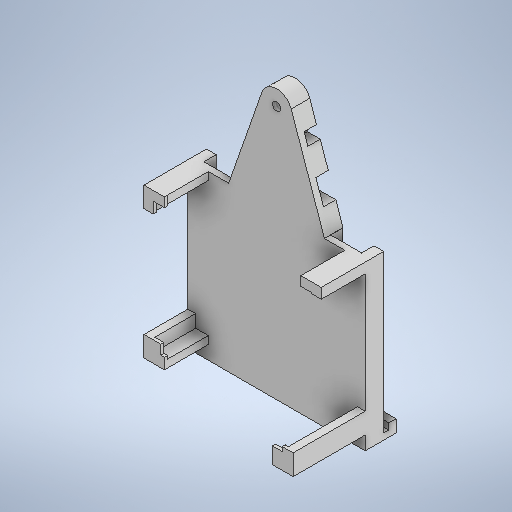
# Autodesk Inventor part: SEN5X_Mount
Saved by Autodesk Inventor 2025 (Build 290162010, 162A)
## iProperties
Created: 2024-07-08
Part Number: SEN5X_Mount
Material: Generic
Document SubType Name: Modeling
Designer: vncnt
Density: 1 g/cm^3
Appearance: Default
Author: vncnt
## iProperties of the stored document SEN5X_Mount_3DPrint.ipt
Created: 2024-07-08
Part Number: SEN5X_Mount_3DPrint
Material: Generic
Document SubType Name: Modeling
Designer: vncnt
Density: 1 g/cm^3
Appearance: Default
Author: vncnt
Autodesk Inventor part; units mm, degrees
ref_plane "YZ Plane" through (0, 0, 0) normal (1, 0, 0) x (0, 1, 0)
ref_plane "XZ Plane" through (0, 0, 0) normal (0, 1, 0) x (-1, 0, 0)
ref_plane "XY Plane" through (0, 0, 0) normal (0, 0, 1) x (1, 0, 0)
sketch "Sketch1" plane through (0, 0, 0) normal (0, 0, 1) x (1, 0, 0)
  line L0 (-28.65, -41.095) -> (28.65, -41.095)
  line L1 (28.65, -41.095) -> (28.65, 11.845)
  line L2 (-28.65, 11.755) -> (-28.65, -41.095)
  line L3 (-28.65, -41.095) -> (28.65, 41.095) construction
  line L4 (28.65, -41.095) -> (-28.65, 41.095) construction
  circle A0 centre (0, 41.005) radius 5
  line L5 (-8.6158, 11.755) -> (12.08, 11.755)
  line L6 (12.08, 11.755) -> (27.305, 11.755)
  line L7 (-8.6158, 11.755) -> (-27.305, 11.755)
  line L8 (-4.7214, 42.6506) -> (-15.49, 11.755)
  line L9 (4.7214, 42.6506) -> (15.49, 11.755)
  line L10 (28.65, -41.095) -> (-28.65, -41.095)
  line L11 (-28.65, -41.095) -> (-28.65, 11.755)
  line L12 (-28.65, 11.755) -> (28.65, 11.755)
  line L13 (28.65, 11.755) -> (28.65, -41.095)
  point P0 (0, 0)
  point P1 (15.49, 11.755)
  point P2 (28.65, -14.625)
  point P3 (28.65, 11.755)
  dimension "d2" = 10
  dimension "d3" = 29.25
  dimension "d26" = 30.98
  dimension "d27" = 15.49
  dimension "d28" = 0
  dimension "d112" = 57.3
  dimension "d113" = 28.65
  dimension "d114" = 82.1
  constraints: 28 end point, 3 horizontal, 3 midpoint, 3 parallel, 3 perpendicular, 2 point on circle, 2 tangent, 1 centre point
  measures "d2" diameter of A0
  measures "d3" distance from line of L5 A0.centre
  measures "d26" distance of L9.end L8.end
  measures "d27" horizontal distance of A0.centre L8.end
  measures "d28" horizontal distance of point (0, 0) A0.centre
  measures "d112" distance from line of point (28.65, -14.625) L2
  measures "d113" distance from line of L2 A0.centre
  measures "d114" distance from line of L0 A0.centre
extrude "Extrusion1" add sketch "Sketch1" along normal blind 2
sketch "Sketch2" plane through (0, 0, 0) normal (0, 0, -1) x (-1, 0, 0)
  arc A0 (4.7214, 42.6506) -> (-4.7214, 42.6506) centre (0, 41.005) ccw projected
  line L0 (28.65, -41.095) -> (-28.65, -41.095) projected
  line L1 (-25.5, -41.095) -> (-15.4, -41.095)
  line L2 (-15.4, -41.095) -> (-15.4, 11.755)
  line L3 (-15.4, 11.755) -> (-25.5, 11.755)
  line L4 (-25.5, 11.755) -> (-25.5, -41.095)
  line L5 (-11.25, -41.095) -> (0, -41.095)
  line L6 (0, -41.095) -> (0, 11.755)
  line L7 (0, 11.755) -> (-11.25, 11.755)
  line L8 (-11.25, 11.755) -> (-11.25, -41.095)
  line L9 (-28.65, -41.095) -> (28.65, -41.095)
  line L10 (15.4, -41.095) -> (15.4, 11.755)
  line L11 (15.4, 11.755) -> (25.5, 11.755)
  line L12 (25.5, 11.755) -> (25.5, -41.095)
  line L13 (0, 11.755) -> (11.25, 11.755)
  line L14 (11.25, 11.755) -> (11.25, -41.095)
  line L15 (0.325, 18.455) -> (0.325, 25.455)
  line L16 (3.4342, 23.4666) -> (3.4342, 16.3794)
  line L17 (-8.1182, 32.905) -> (-3.965, 32.905)
  line L18 (-3.965, 32.905) -> (-3.965, 36.405)
  line L19 (-3.965, 36.405) -> (-6.8983, 36.405)
  line L20 (-9.0424, 34.1387) -> (-3.965, 36.405) construction
  line L21 (-3.965, 32.905) -> (-8.76, 36.4299) construction
  line L22 (2.695, 38.3741) -> (6.212, 38.3741)
  line L23 (2.695, 38.3741) -> (6.195, 41.0959) construction
  line L24 (9.0035, 30.365) -> (5.235, 30.365)
  line L25 (5.235, 30.365) -> (5.235, 33.865)
  line L26 (5.235, 33.865) -> (7.7836, 33.865)
  line L27 (10.412, 31.3708) -> (5.235, 33.865) construction
  line L28 (5.235, 30.365) -> (10.1967, 33.5777) construction
  line L29 (11.2334, 23.4684) -> (11.4073, 23.4684)
  line L30 (-27.305, 11.755) -> (-15.49, 11.755)
  line L31 (28.65, -41.095) -> (-28.65, -41.095)
  line L32 (-27.305, 11.755) -> (28.65, 11.755)
  line L33 (28.65, 11.755) -> (28.65, -41.095)
  line L34 (-15.49, 11.755) -> (-4.7214, 42.6506) projected
  line L35 (4.7214, 42.6506) -> (15.49, 11.755) projected
  line L36 (-15.49, 11.755) -> (-13.0996, 18.6131)
  line L37 (15.49, 11.755) -> (13.9048, 16.3032)
  line L38 (11.4073, 23.4684) -> (8.8839, 30.7082)
  line L39 (8.3097, 32.3558) -> (8.298, 32.3893)
  line L40 (7.732, 34.0131) -> (6.1901, 38.437)
  line L41 (5.1818, 41.3299) -> (4.7214, 42.6506)
  line L42 (-10.6022, 25.7784) -> (-7.4388, 34.8545)
  line L43 (-7.2711, 35.3354) -> (-4.7214, 42.6506)
  arc A1 (6.1415, 38.3741) -> (6.1901, 38.437) centre (4.445, 39.735) ccw
  arc A2 (2.695, 39.735) -> (2.6956, 39.6883) centre (4.445, 39.735) ccw
  arc A3 (4.7214, 42.6506) -> (-4.7214, 42.6506) centre (0, 41.005) ccw
  arc A4 (2.695, 39.6871) -> (2.6956, 39.6883) centre (0, 41.005) ccw
  line L44 (-27.305, 11.755) -> (-15.49, 11.755)
  line L45 (-28.65, -39.095) -> (28.65, -39.095)
  line L46 (-25.5, 11.755) -> (-28.65, 11.755)
  line L47 (-28.65, 11.755) -> (-28.65, -39.095)
  line L48 (-28.65, -39.095) -> (-25.5, -39.095)
  line L49 (-25.5, -39.095) -> (-25.5, 11.755)
  line L50 (-28.65, -39.095) -> (-28.65, -41.095)
  line L51 (2.695, 38.3741) -> (6.195, 38.3741)
  line L52 (6.195, 38.3741) -> (6.195, 47.1002)
  line L53 (6.195, 47.1002) -> (2.695, 47.1002)
  line L54 (2.695, 47.1002) -> (2.695, 38.3741)
  line L55 (3.4342, 23.4666) -> (15.1988, 23.4666)
  line L56 (15.1988, 23.4666) -> (15.1988, 16.4666)
  line L57 (15.1988, 16.4666) -> (3.4342, 16.4666)
  line L58 (3.4342, 16.4666) -> (3.4342, 23.4666)
  line L59 (0.325, 25.455) -> (-14.4798, 25.455)
  line L60 (-14.4798, 25.455) -> (-14.4798, 18.455)
  line L61 (-14.4798, 18.455) -> (0.325, 18.455)
  line L62 (0.325, 18.455) -> (0.325, 25.455)
  point P0 (0, 0)
  point P1 (4.9516, 41.9903)
  point P2 (5.235, 32.115)
  point P3 (-3.965, 34.655)
  point P4 (2.695, 44.9696)
  point P5 (0.325, 21.955)
  point P6 (3.4342, 19.923)
  point P7 (11.25, -41.095)
  point P8 (15.4, -41.095)
  point P9 (25.5, -41.095)
  point P10 (28.65, -41.095)
  point P11 (9.0035, 30.365)
  point P12 (6.212, 38.3741)
  point P13 (-25.5, -41.095)
  point P14 (-15.4, 11.755)
  point P15 (15.49, 11.755)
  point P16 (-15.4, 11.755)
  point P17 (-15.4, -41.095)
  point P18 (-11.25, -41.095)
  point P19 (6.1901, 38.437)
  point P20 (2.6952, 39.7117)
  point P21 (-15.4, -39.095)
  point P22 (-25.5, -39.095)
  point P23 (25.5, -39.095)
  point P24 (15.4, -39.095)
  point P25 (-11.25, -39.095)
  point P26 (11.25, -39.095)
  point P27 (6.9533, 34.0365)
  point P28 (2.695, 39.735)
  point P29 (2.695, 45.2165)
  point P30 (-10.7149, 25.455)
  point P31 (-13.1547, 18.455)
  point P32 (13.8478, 16.4666)
  point P33 (3.4342, 16.4666)
  point P34 (10.829, 23.4666)
  point P35 (11.408, 23.4666)
  point P36 (4.445, 38.3741)
  dimension "d22" = 25.5
  dimension "d23" = 15.4
  dimension "d24" = 11.25
  dimension "d25" = 11.25
  dimension "d38" = 19.05
  dimension "d44" = 3.965
  dimension "d45" = 5.235
  dimension "d46" = 0.325
  dimension "d47" = 3.4342
  dimension "d48" = 21.082
  dimension "d49" = 8.89
  dimension "d50" = 6.35
  dimension "d51" = 2
  dimension "d138" = 7
  dimension "d139" = 7
  dimension "d140" = 3.5
  dimension "d141" = 3.5
  dimension "d142" = 3.5
  dimension "d143" = 4.445
  dimension "d144" = 1.27
  constraints: 120 end point, 22 point on line, 15 parallel, 11 horizontal, 11 tangent, 10 perpendicular, 9 point on circle, 8 collinear, 8 symmetric about line, 7 midpoint, 4 centre point, 2 coincident
  measures "d22" distance from line of L4 point (0, 0)
  measures "d23" distance from line of L2 point (0, 0)
  measures "d24" distance of L6.end L7.end
  measures "d25" distance from line of L8 point (0, 0)
  measures "d38" vertical distance of point (0.325, 21.955) A3.centre
  measures "d44" horizontal distance of point (-3.965, 34.655) A0.centre
  measures "d45" horizontal distance of point (5.235, 32.115) A0.centre
  measures "d46" distance from line of L15 A0.centre
  measures "d47" horizontal distance of A0.centre point (3.434, 19.923)
  measures "d48" vertical distance of A0.centre point (3.434, 19.923)
  measures "d49" vertical distance of point (5.235, 32.115) A0.centre
  measures "d50" vertical distance of point (-3.965, 34.655) A0.centre
  measures "d51" distance between parallel lines of L0 L45
  measures "d138" distance between parallel lines of L61 L59
  measures "d139" distance between parallel lines of L57 L55
  measures "d140" distance between parallel lines of L17 L19
  measures "d141" distance between parallel lines of L24 L26
  measures "d142" distance between parallel lines of L52 L54
  measures "d143" horizontal distance of point (4.445, 38.374) A0.centre
  measures "d144" vertical distance of A0.centre A1.centre
extrude "Extrusion2" add sketch "Sketch2" along normal blind 4 contours L54 A4 L22 L35 L26 L25 L24 L29 L55 L16 L57 L11 L32 L13 L7 L3 L34 L61 L15 L59 L17 L18 L19 A0 | L54 A2 A4 | L35 L52 L22 A1 | L35 L22 L52 | L32 L8 L45 L2 | L4 L45 L47 L46 L30 | L45 L8 L0 L2 | L2 L0 L4 L45 | L4 L0 L50 L45 | L45 L6 L0 L8 | L10 L45 L14 L32 | L32 L33 L45 L12 | L45 L14 L0 L6 | L45 L12 L0 L10 | L10 L0 L14 L45 | L45 L33 L0 L12 picked at (-0.9552, 41.2924)
sketch "Sketch3" plane through (0, 0, 2) normal (0, 0, 1) x (1, 0, 0)
  line L0 (-15.49, 11.755) -> (-28.65, 11.755)
  line L1 (28.65, -41.095) -> (28.65, 11.755) projected
  line L2 (-28.65, 11.755) -> (28.65, 11.755)
  line L3 (28.65, 11.755) -> (28.65, -41.095)
  line L4 (37.294, -28.9953) -> (-37.344, 8.455) construction
  line L5 (20.655, -45.4719) -> (-20.705, 24.9315) construction
  line L6 (-28.65, 11.755) -> (-22.05, 11.755)
  line L7 (-22.05, 11.755) -> (-22.05, 5.155)
  line L8 (-22.05, 5.155) -> (-28.65, 5.155)
  line L9 (-28.65, 5.155) -> (-28.65, 11.755)
  line L10 (28.65, 11.755) -> (22.05, 11.755)
  line L11 (22.05, 11.755) -> (22.05, 8.455)
  line L12 (22.05, 8.455) -> (28.65, 8.455)
  line L13 (28.65, 8.455) -> (28.65, 11.755)
  line L14 (-22.05, 5.155) -> (-26.15, 5.155)
  line L15 (-26.15, 5.155) -> (-26.15, 9.255)
  line L16 (-26.15, 9.255) -> (-22.05, 9.255)
  line L17 (-22.05, 9.255) -> (-22.05, 5.155)
  line L18 (22.05, 8.455) -> (26.15, 8.455)
  line L19 (26.15, 8.455) -> (26.15, 9.255)
  line L20 (26.15, 9.255) -> (22.05, 9.255)
  line L21 (22.05, 9.255) -> (22.05, 8.455)
  line L22 (22.05, 8.455) -> (25.65, 8.455)
  line L23 (22.05, 8.755) -> (22.05, 8.455)
  line L24 (-28.65, 11.755) -> (-28.65, -41.095) projected
  line L25 (-28.65, -36.665) -> (-22.05, -36.665)
  line L26 (-22.05, -36.665) -> (-22.05, -30.065)
  line L27 (-22.05, -30.065) -> (-28.65, -30.065)
  line L28 (-28.65, -30.065) -> (-28.65, -36.665)
  line L29 (-22.05, -30.065) -> (-26.15, -30.065)
  line L30 (-26.15, -30.065) -> (-26.15, -34.165)
  line L31 (-26.15, -34.165) -> (-22.05, -34.165)
  line L32 (-22.05, -34.165) -> (-22.05, -30.065)
  point P0 (0, 0)
  point P1 (27.305, 11.755)
  point P2 (-22.07, 11.755)
  point P3 (24.305, 8.605)
  point P4 (28.65, 8.455)
  point P5 (27.305, 11.755)
  point P6 (22.05, 11.755)
  point P7 (-22.05, 11.755)
  point P8 (-24.1, 9.255)
  point P9 (-28.65, -30.065)
  dimension "d58" = 6.6
  dimension "d59" = 6.6
  dimension "d60" = 6.6
  dimension "d61" = 3.3
  dimension "d63" = 2.5
  dimension "d69" = 2.5
  dimension "d70" = 2.5
  dimension "d100" = 6.6
  dimension "d101" = 6.6
  dimension "d102" = 2.5
  dimension "d103" = 2.5
  dimension "d104" = 43.42
  dimension "d115" = 2.5
  constraints: 62 end point, 12 parallel, 8 horizontal, 7 perpendicular, 2 midpoint, 1 point on line, 1 other
  measures "d58" distance of L7.end L8.end
  measures "d59" distance of L6.end L7.end
  measures "d60" distance of L12.end L11.end
  measures "d61" distance of L11.end L10.end
  measures "d63" distance between parallel lines of L0 L16
  measures "d69" distance between parallel lines of L2 L20
  measures "d70" distance between parallel lines of L3 L19
  measures "d100" distance of L25.end L26.end
  measures "d101" distance of L25.start L25.end
  measures "d102" distance between parallel lines of L25 L31
  measures "d103" distance between parallel lines of L24 L30
  measures "d104" distance between parallel lines of L16 L31
  measures "d115" distance between parallel lines of L24 L15
extrude "Extrusion3" add sketch "Sketch3" along normal blind 13.207 contours L7 L16 L15 L8 L9 L0 | L12 L19 L20 L11 L2 L1 | L27 L30 L31 L26 L25 L24
sketch "Sketch4" plane through (0, 0, 2) normal (0, 0, 1) x (1, 0, 0)
  line L0 (28.65, -41.095) -> (28.65, 8.455) projected
  line L1 (28.65, -36.665) -> (22, -36.665)
  line L2 (22, -36.665) -> (22, -30.015)
  line L3 (22, -30.015) -> (28.65, -30.015)
  line L4 (28.65, -30.015) -> (28.65, -41.095)
  line L5 (22, -30.015) -> (26.15, -30.015)
  line L6 (26.15, -30.015) -> (26.15, -34.165)
  line L7 (26.15, -34.165) -> (22, -34.165)
  line L8 (22, -34.165) -> (22, -30.015)
  point P0 (0, 0)
  point P1 (25.325, -36.665)
  point P2 (22.05, 9.255)
  point P3 (28.65, -36.665)
  dimension "d75" = 6.65
  dimension "d76" = 6.65
  dimension "d77" = 2.5
  dimension "d78" = 2.5
  dimension "d97" = 43.42
  constraints: 16 end point, 4 parallel, 2 horizontal, 1 midpoint, 1 perpendicular
  measures "d75" distance of L1.start L1.end
  measures "d76" distance between parallel lines of L1 L3
  measures "d77" distance between parallel lines of L0 L6
  measures "d78" distance from line of point (25.325, -36.665) L7
  measures "d97" distance of L7.end point (22.05, 9.255)
extrude "Extrusion4" add sketch "Sketch4" along normal blind 22.3 contours L1 L2 L7 L6 L3 L0
sketch "Sketch5" plane through (0, 0, 15.207) normal (0, 0, 1) x (1, 0, 0)
  line L0 (-28.65, 11.755) -> (-25.5, 11.755)
  line L1 (-28.65, 11.755) -> (-22.046, 11.755)
  line L2 (-22.046, 11.755) -> (-22.046, 5.151)
  line L3 (-22.046, 5.151) -> (-28.65, 5.151)
  line L4 (-28.65, 5.151) -> (-28.65, 11.755)
  line L5 (-22.046, 5.151) -> (-25.65, 5.151)
  line L6 (-25.65, 5.151) -> (-25.65, 8.755)
  line L7 (-25.65, 8.755) -> (-22.046, 8.755)
  line L8 (-22.046, 8.755) -> (-22.046, 5.151)
  line L9 (-26.15, 9.255) -> (-22.05, 9.255)
  line L10 (-26.15, 5.155) -> (-26.15, 9.255)
  line L11 (28.65, 11.755) -> (22.05, 11.755)
  line L12 (22.05, 11.755) -> (22.05, 8.453)
  line L13 (22.05, 8.453) -> (28.65, 8.453)
  line L14 (28.65, 8.453) -> (28.65, 11.755)
  line L15 (22.05, 8.453) -> (25.65, 8.453)
  line L16 (25.65, 8.453) -> (25.65, 8.755)
  line L17 (25.65, 8.755) -> (22.05, 8.755)
  line L18 (22.05, 8.755) -> (22.05, 8.453)
  line L19 (22.05, 9.255) -> (26.15, 9.255)
  line L20 (26.15, 9.255) -> (26.15, 8.455)
  line L21 (-28.65, -30.065) -> (-26.15, -30.065)
  line L22 (-28.65, -36.665) -> (-22.05, -36.665) projected
  line L23 (-28.65, -30.065) -> (-22.05, -30.065)
  line L24 (-22.05, -30.065) -> (-22.05, -36.665)
  line L25 (-22.05, -36.665) -> (-28.65, -36.665)
  line L26 (-28.65, -36.665) -> (-28.65, -30.065)
  line L27 (-22.05, -30.065) -> (-23.25, -30.065)
  line L28 (-23.25, -30.065) -> (-23.25, -33.165)
  line L29 (-23.25, -33.165) -> (-22.05, -33.165)
  line L30 (-22.05, -33.165) -> (-22.05, -30.065)
  line L31 (-28.65, -36.665) -> (-22.05, -36.665)
  point P0 (0, 0)
  point P1 (-26.15, 7.205)
  dimension "d81" = 6.604
  dimension "d82" = 6.604
  dimension "d83" = 0.5
  dimension "d84" = 0.5
  dimension "d87" = 0.5
  dimension "d88" = 0.5
  dimension "d105" = 3.5
  dimension "d106" = 5.4
  constraints: 62 end point, 13 equal length, 6 horizontal, 6 perpendicular, 1 coincident, 1 midpoint
  measures "d81" distance of L2.end L3.end
  measures "d82" distance of L1.end L2.end
  measures "d83" distance between parallel lines of L7 L9
  measures "d84" distance from line of point (-26.15, 7.205) L6
  measures "d87" distance between parallel lines of L19 L17
  measures "d88" distance between parallel lines of L20 L16
  measures "d105" distance between parallel lines of L22 L29
  measures "d106" distance between parallel lines of L26 L28
extrude "Extrusion5" add sketch "Sketch5" along normal blind 1 contours L0 L1 L2 L7 L6 L3 L4 | L14 L13 L20 L19 L12 L11 | L19 L20 L13 L16 L17 L12 | L21 L23 L28 L29 L24 L22 L26
sketch "Sketch6" plane through (0, 0, 24.3) normal (0, 0, 1) x (1, 0, 0)
  line L0 (26.15, -30.015) -> (28.65, -30.015) projected
  line L1 (22, -36.665) -> (22, -34.165) projected
  line L2 (28.65, -30.015) -> (22, -30.015)
  line L3 (21.7942, -36.665) -> (28.4442, -36.665)
  line L4 (28.65, -41.005) -> (28.65, -30.015)
  line L5 (22, -30.015) -> (25.15, -30.015)
  line L6 (25.15, -30.015) -> (25.15, -31.395)
  line L7 (25.15, -31.395) -> (22, -31.395)
  line L8 (22, -31.395) -> (22, -30.015)
  line L9 (22, -36.665) -> (28.65, -36.665) projected
  line L10 (22, -31.395) -> (22, -36.665)
  point P0 (0, 0)
  point P1 (20.655, -31.395)
  point P2 (23.805, -30.015)
  dimension "d93" = 5.27
  dimension "d94" = 3.5
  constraints: 16 end point, 3 perpendicular, 2 horizontal, 2 parallel
  measures "d93" distance between parallel lines of L3 L7
  measures "d94" distance between parallel lines of L4 L6
extrude "Extrusion6" add sketch "Sketch6" along normal blind 1 contours L0 L4 L9 L3 L1 L10 L7 L6 L2
sketch "Sketch9" plane through (28.65, -41.095, -4) normal (1, 0, 0) x (0, 0, -1)
  line L0 (0, 0) -> (-6, 0) projected
  line L1 (0, 0) -> (4, 0)
  line L2 (4, 0) -> (4, 4)
  line L3 (4, 4) -> (0, 4)
  line L4 (0, 4) -> (0, 0)
  line L5 (0, 2) -> (4, 2)
  line L6 (4, 2) -> (4, 0)
  line L7 (4, 0) -> (0, 0)
  line L8 (0, 0) -> (0, 2)
  line L9 (4, 2) -> (1.66, 2)
  line L10 (1.66, 2) -> (1.66, 4)
  line L11 (1.66, 4) -> (4, 4)
  line L12 (4, 4) -> (4, 2)
  point P0 (-4, 41.095)
  point P1 (1.66, 2)
  dimension "d116" = 1.66
  dimension "d118" = 4
  dimension "d119" = 2
  constraints: 24 end point, 6 parallel, 3 horizontal, 3 perpendicular, 1 point on line
  measures "d116" distance between parallel lines of L4 L10
  measures "d118" distance between parallel lines of L2 L4
  measures "d119" distance between parallel lines of L5 L3
extrude "Extrusion8" add sketch "Sketch9" against normal up to surface (57.3 mm away) contours L4 L5 L2 L1 | L5 L10 L3 L2
sketch "Sketch11" plane through (0, 0, 2) normal (0, 0, 1) x (1, 0, 0)
  arc A0 (4.7214, 42.6506) -> (-4.7214, 42.6506) centre (0, 41.005) ccw projected
  point P0 (0, 0)
  constraints: 1 coincident
hole "Hole1" at (0, 41.005, 2) direction (0, 0, -1) diameter 2.6416 depth 10.979 thread size "6-32 UNC" class "2B" standard "ANSI Unified Screw Threads"
sketch "Sketch15" plane through (28.65, -41.095, -8) normal (0, 0, -1) x (-1, 0, 0)
  line L0 (17.4, 2) -> (17.4, 52.85) projected
  line L1 (39.9, 2) -> (39.9, 52.85) projected
  line L2 (39.9, 2) -> (39.9, 24.2039)
  line L3 (39.9, 24.2039) -> (17.4, 24.2039)
  line L4 (17.4, 24.2039) -> (17.4, 2)
  line L5 (39.9, 2) -> (39.9, -3.1945)
  line L6 (39.9, -3.1945) -> (17.4, -3.1945)
  line L7 (17.4, -3.1945) -> (17.4, 2)
  point P0 (28.65, 41.095)
  point P1 (17.4, 24.2039)
  constraints: 12 end point, 2 parallel, 1 point on line
extrude "Extrusion13" cut sketch "Sketch15" against normal up to surface (8 mm away)
body "Solid1"
